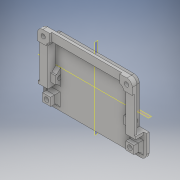
# Autodesk Inventor part: case_back
Saved by Autodesk Inventor 2018 (Build 220112000, 112)
## iProperties
Created: 2018-08-02
Part Number: case_back
Material: Generic
Document SubType Name: Modeling
Designer: Luke
Density: 1 g/cm^3
Appearance: Default
Author: Luke
Autodesk Inventor part; units mm, degrees
ref_plane "YZ Plane" through (0, 0, 0) normal (1, 0, 0) x (0, 1, 0)
ref_plane "XZ Plane" through (0, 0, 0) normal (0, 1, 0) x (-1, 0, 0)
ref_plane "XY Plane" through (0, 0, 0) normal (0, 0, 1) x (1, 0, 0)
sketch "Sketch1" plane through (0, 0, 0) normal (0, 1, 0) x (-1, 0, 0)
  line L0 (0, 0) -> (-76.5, 0)
  line L1 (-76.5, 0) -> (-76.5, 56.5)
  line L2 (-76.5, 56.5) -> (0, 56.5)
  line L3 (0, 56.5) -> (0, 0)
  dimension "d0" = 76.5
  dimension "d1" = 56.5
  constraints: 8 end point, 2 parallel, 1 horizontal, 1 perpendicular
  measures "d0" distance of L0.start L0.end
  measures "d1" distance of L0.end L1.end
extrude "Extrusion1" add sketch "Sketch1" along normal blind 2
ref_plane "Work Plane1" through (0, 0, 28.25) normal (0, 0, 1) x (1, 0, 0)
ref_plane "Work Plane2" through (38.25, 0, 0) normal (-1, 0, 0) x (0, 0, 1)
sketch "Sketch2" plane through (0, 2, 0) normal (0, 1, 0) x (1, 0, 0)
  line L0 (38.25, -67.8) -> (38.25, 11.3) construction
  line L1 (91.8, -28.25) -> (-15.3, -28.25) construction
  line L2 (7.25, -7.25) -> (69.25, -7.25) construction
  line L3 (69.25, -7.25) -> (69.25, -49.25) construction
  line L4 (69.25, -49.25) -> (7.25, -49.25) construction
  line L5 (7.25, -49.25) -> (7.25, -7.25) construction
  circle A0 centre (7.25, -7.25) radius 1.75
  circle A1 centre (69.25, -7.25) radius 1.75
  point P0 (0, 0)
  dimension "d4" = 62
  dimension "d5" = 42
  dimension "d6" = 3.5
  dimension "d7" = 3.5
  constraints: 8 end point, 2 centre point, 2 coincident, 2 parallel, 1 horizontal, 1 perpendicular, 2 other
  measures "d4" distance of L2.start L2.end
  measures "d5" distance of L2.end L3.end
  measures "d6" diameter of A0
  measures "d7" diameter of A1
sketch "Sketch3" plane through (0, 2, 0) normal (0, 1, 0) x (1, 0, 0)
  line L0 (76.5, 0) -> (0, 0) projected
  line L1 (0, 0) -> (0, -56.5) projected
  line L2 (0, -56.5) -> (76.5, -56.5) projected
  line L3 (76.5, -56.5) -> (76.5, 0) projected
  line L4 (0, -56.5) -> (0, 0) projected
  line L5 (0, -17.5) -> (7.25, -17.5)
  line L6 (7.25, -17.5) -> (7.25, -49.5)
  line L7 (7.25, -49.5) -> (69.25, -49.5)
  line L8 (69.25, -49.5) -> (69.25, -17.5)
  line L9 (69.25, -17.5) -> (76.5, -17.5)
  line L10 (38.25, -67.8) -> (38.25, 11.3) construction
  dimension "d12" = 62
  dimension "d13" = 7
  dimension "d14" = 39
  constraints: 10 end point, 4 perpendicular, 4 point on line, 1 other
  measures "d12" distance of L6.end L7.end
  measures "d13" distance between parallel lines of L2 L7
  measures "d14" distance between parallel lines of L2 L5
extrude "Extrusion3" cut sketch "Sketch3" against normal up to surface (2 mm away) contours L3 L2 L1 L5 L6 L7 L8 L9
extrude "Extrusion4" cut sketch "Sketch2" against normal up to surface (2 mm away)
sketch "Sketch4" plane through (0, 0, 0) normal (0, -1, 0) x (1, 0, 0)
  line L0 (7.25, 17.5) -> (0, 17.5) projected
  line L1 (7.25, 49.5) -> (7.25, 17.5) projected
  line L2 (69.25, 49.5) -> (7.25, 49.5) projected
  line L3 (69.25, 17.5) -> (69.25, 49.5) projected
  line L4 (76.5, 17.5) -> (69.25, 17.5) projected
  line L5 (0, 17.5) -> (0, 0) projected
  line L6 (76.5, 0) -> (76.5, 17.5) projected
  line L7 (9.25, 15.5) -> (9.25, 47.5)
  line L8 (9.25, 47.5) -> (67.25, 47.5)
  line L9 (67.25, 47.5) -> (67.25, 15.5)
  line L10 (67.25, 15.5) -> (74.5, 15.5)
  line L11 (74.5, 15.5) -> (74.5, 17.5)
  line L12 (69.25, 17.5) -> (76.5, 17.5) projected
  line L13 (9.25, 15.5) -> (2, 15.5)
  line L14 (2, 15.5) -> (2, 17.5)
  dimension "d20" = 2
  dimension "d21" = 2
  dimension "d22" = 2
  dimension "d25" = 2
  dimension "d26" = 2
  dimension "d27" = 2
  constraints: 14 end point, 4 perpendicular, 2 horizontal, 2 point on line, 1 collinear
  measures "d20" distance between parallel lines of L3 L9
  measures "d21" distance between parallel lines of L2 L8
  measures "d22" distance between parallel lines of L1 L7
  measures "d25" distance between parallel lines of L5 L14
  measures "d26" distance between parallel lines of L6 L11
  measures "d27" distance between parallel lines of L4 L10
extrude "Extrusion5" add sketch "Sketch4" along normal blind 4
sketch "Sketch5" plane through (69.25, 2, 49.5) normal (1, 0, 0) x (0, 0, -1)
  line L0 (32, 0) -> (32, -6) construction
  line L1 (0, 0) -> (32, 0) construction
  line L2 (0, 0) -> (0, -6) construction
  line L3 (32, -6) -> (0, -6) construction
  circle A0 centre (27.5, -2.75) radius 1.6
  point P0 (49.5, -2)
  dimension "d28" = 3.2
  dimension "d29" = 2.75
  dimension "d30" = 4.5
  constraints: 1 centre point
  measures "d28" diameter of A0
  measures "d29" distance from line of L1 A0.centre
  measures "d30" distance from line of L0 A0.centre
extrude "Extrusion6" cut sketch "Sketch5" against normal up to surface (2 mm away)
sketch "Sketch6" plane through (67.25, -4, 15.5) normal (-1, 0, 0) x (0, 0, 1)
  arc A0 (5.0867, 4) -> (7.9133, 4) centre (6.5, 3.25) ccw projected
  line L0 (0, 4) -> (5.0867, 4) projected
  line L1 (7.9133, 4) -> (32, 4) projected
  line L2 (9.5, 4) -> (3.5, 4)
  line L3 (3.5, 4) -> (3.5, 0)
  line L4 (3.5, 0) -> (9.5, 0)
  line L5 (9.5, 0) -> (9.5, 4)
  line L6 (6.5, 3.25) -> (6.5, 4) construction
  point P0 (-15.5, 4)
  dimension "d33" = 6
  dimension "d34" = 4
  constraints: 10 end point, 2 parallel, 2 perpendicular, 1 horizontal, 1 midpoint, 1 point on line, 1 other
  measures "d33" distance of L3.end L4.end
  measures "d34" distance of L2.end L3.end
extrude "Extrusion7" add sketch "Sketch6" along normal blind 3.5
sketch "Sketch7" plane through (67.25, -0.75, 22) normal (1, 0, 0) x (0, 0, -1)
  circle A0 centre (0, 0) radius 1.6 projected
  point P0 (22, 0.75)
extrude "Extrusion8" cut sketch "Sketch7" against normal up to surface (3.5 mm away)
sketch "Sketch8" plane through (0, -4, 0) normal (0, -1, 0) x (1, 0, 0)
  line L0 (7.25, 17.5) -> (2, 17.5) projected
  line L1 (2, 17.5) -> (2, 15.5) projected
  line L2 (2, 15.5) -> (9.25, 15.5) projected
  line L3 (9.25, 15.5) -> (9.25, 47.5) projected
  line L4 (9.25, 47.5) -> (67.25, 47.5) projected
  line L5 (67.25, 47.5) -> (67.25, 25) projected
  line L6 (67.25, 15.5) -> (74.5, 15.5) projected
  line L7 (74.5, 15.5) -> (74.5, 17.5) projected
  line L8 (74.5, 17.5) -> (69.25, 17.5) projected
  line L9 (69.25, 17.5) -> (69.25, 49.5) projected
  line L10 (69.25, 49.5) -> (7.25, 49.5) projected
  line L11 (7.25, 49.5) -> (7.25, 17.5) projected
  line L12 (73.5, 17.5) -> (73.5, 53.5)
  line L13 (73.5, 53.5) -> (3, 53.5)
  line L14 (3, 53.5) -> (3, 17.5)
  line L15 (74.5, 17.5) -> (69.25, 17.5) projected
  line L16 (7.25, 17.5) -> (2, 17.5) projected
  line L17 (67.25, 25) -> (63.75, 25) construction
  line L18 (63.75, 19) -> (63.75, 25) construction
  line L19 (67.25, 19) -> (63.75, 19) construction
  line L20 (67.25, 19) -> (67.25, 15.5) projected
  line L21 (67.25, 25) -> (67.25, 19)
  point P0 (0, 0)
  dimension "d39" = 53.5
  dimension "d65" = 1
  dimension "d66" = 1
  constraints: 8 end point, 2 perpendicular, 2 point on line, 2 vertical
  measures "d39" distance from line of L13 point (0, 0)
  measures "d65" distance between parallel lines of L1 L14
  measures "d66" distance between parallel lines of L12 L7
extrude "Extrusion9" add sketch "Sketch8" along normal blind 2
fillet "Fillet1" radius 4 4 edges at (0, 1, 0) (76.5, 1, 0) (3, -5, 53.5) (73.5, -5, 53.5)
fillet "Fillet2" radius 4 4 edges at (7.25, -1, 49.5) (69.25, -1, 49.5) (9.25, -3, 47.5) (67.25, -3, 47.5)
sketch "Sketch9" plane through (0, 0, 0) normal (0, -1, 0) x (1, 0, 0)
  circle A0 centre (69.25, 7.25) radius 1.75 projected
  circle A1 centre (7.25, 7.25) radius 1.75 projected
  line L0 (72.25, 10.25) -> (66.25, 10.25)
  line L1 (66.25, 10.25) -> (66.25, 4.25)
  line L2 (66.25, 4.25) -> (72.25, 4.25)
  line L3 (72.25, 4.25) -> (72.25, 10.25)
  line L4 (72.25, 10.25) -> (66.25, 4.25) construction
  line L5 (66.25, 10.25) -> (72.25, 4.25) construction
  line L6 (10.25, 10.25) -> (4.25, 10.25)
  line L7 (4.25, 10.25) -> (4.25, 4.25)
  line L8 (4.25, 4.25) -> (10.25, 4.25)
  line L9 (10.25, 4.25) -> (10.25, 10.25)
  line L10 (10.25, 10.25) -> (4.25, 4.25) construction
  line L11 (4.25, 10.25) -> (10.25, 4.25) construction
  point P0 (0, 0)
  dimension "d44" = 6
  dimension "d45" = 6
  dimension "d46" = 6
  dimension "d47" = 6
  constraints: 24 end point, 4 midpoint, 4 parallel, 2 horizontal, 2 perpendicular
  measures "d44" distance of L1.end L2.end
  measures "d45" distance of L0.end L1.end
  measures "d46" distance of L8.end L6.start
  measures "d47" distance of L7.end L8.end
extrude "Extrusion10" add sketch "Sketch9" along normal blind 5
sketch "Sketch10" plane through (0, 2, 0) normal (0, 1, 0) x (1, 0, 0)
  circle A0 centre (69.25, -7.25) radius 1.75 projected
  circle A1 centre (7.25, -7.25) radius 1.75 projected
  point P0 (0, 0)
extrude "Extrusion11" add sketch "Sketch10" against normal blind 1
sketch "Sketch11" plane through (0, -4, 0) normal (0, 1, 0) x (1, 0, 0)
  circle A0 centre (7.25, -7.25) radius 1.75 construction
  circle A1 centre (69.25, -7.25) radius 1.75 construction
  circle A2 centre (69.25, -7.25) radius 1.75 construction
  line L0 (7.25, -7.25) -> (69.25, -7.25) construction
  line L1 (69.25, -7.25) -> (69.25, -49.25) construction
  line L2 (69.25, -49.25) -> (7.25, -49.25) construction
  line L3 (7.25, -49.25) -> (7.25, -7.25) construction
  circle A3 centre (7.25, -49.25) radius 1.6
  circle A4 centre (69.25, -49.25) radius 1.6
  point P0 (0, 0)
  dimension "d52" = 3.2
  dimension "d53" = 3.2
  dimension "d54" = 42
  constraints: 8 end point, 3 coincident, 2 centre point, 2 parallel, 1 horizontal, 1 perpendicular
  measures "d52" diameter of A3
  measures "d53" diameter of A4
  measures "d54" distance of L0.end L1.end
extrude "Extrusion12" cut sketch "Sketch11" against normal up to surface (2 mm away)
sketch "Sketch14" plane through (0, -6, 0) normal (0, -1, 0) x (1, 0, 0)
  arc A0 (73.5, 49.5) -> (69.5, 53.5) centre (69.5, 49.5) ccw projected
  line L0 (73.5, 17.5) -> (73.5, 49.5) projected
  line L1 (69.5, 53.5) -> (7, 53.5) projected
  arc A1 (67.25, 43.5) -> (63.25, 47.5) centre (63.25, 43.5) ccw projected
  line L2 (67.25, 43.5) -> (67.25, 15.5) projected
  line L3 (13.25, 47.5) -> (63.25, 47.5) projected
  circle A2 centre (69.25, 49.25) radius 1.6 projected
  line L4 (67.1791, 44.25) -> (73.5, 44.25)
  line L5 (63.25, 47.5) -> (13.25, 47.5) projected
  line L6 (64.25, 47.373) -> (64.25, 53.5)
  line L7 (69.5, 53.5) -> (7, 53.5) projected
  point P0 (0, 0)
  dimension "d67" = 5
  dimension "d68" = 5
  constraints: 4 end point, 2 perpendicular, 2 point on circle, 2 point on line
  measures "d67" distance from line of A2.centre L6
  measures "d68" distance from line of L4 A2.centre
extrude "Extrusion15" add sketch "Sketch14" along normal blind 1.5
sketch "Sketch15" plane through (0, -4, 0) normal (0, 1, 0) x (1, 0, 0)
  arc A0 (67.7939, -48.5868) -> (68.4944, -47.8397) centre (69.25, -49.25) ccw projected
  circle A1 centre (69.25, -49.25) radius 3
  point P0 (0, 0)
  dimension "d71" = 6
  constraints: 1 centre point, 1 coincident
  measures "d71" diameter of A1
extrude "Extrusion16" cut sketch "Sketch15" along normal blind 4
mirror "Mirror2" about plane through (38.25, 0, 0) normal (-1, 0, 0) of "Extrusion16", "Extrusion15"
fillet "Fillet3" radius 2 8 edges at (7.25, 0, 10.25) (4.25, 0, 7.25) (7.25, 0, 4.25) (10.25, 0, 7.25) (69.25, 0, 4.25) (66.25, 0, 7.25) (72.25, 0, 7.25) (69.25, 0, 10.25)
mirror "Mirror4" about plane through (38.25, 0, 0) normal (-1, 0, 0) of "Extrusion6", "Extrusion7", "Extrusion8"
chamfer "Chamfer1" distance 3 angle 45 4 edges at (11, 0, 19) (11, 0, 25) (65.5, 0, 25) (65.5, 0, 19)
sketch "Sketch16" plane through (0, -4, 0) normal (0, 1, 0) x (1, 0, 0)
  circle A0 centre (7.25, -49.25) radius 1.6 projected
  circle A1 centre (69.25, -49.25) radius 1.6 projected
  point P0 (0, 0)
extrude "Extrusion17" [suppressed]
equation "\"d7\" = d6"
equation "\"d21\" = d20"
equation "\"d22\" = d21"
equation "\"d26\" = d25"
equation "\"d45\" = d44"
equation "\"d46\" = d45"
equation "\"d47\" = d45"
equation "\"d68\" = d67"
body "Solid1"
